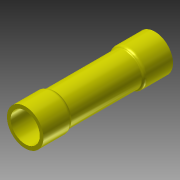
# Autodesk Inventor part: 12-10 double sided female tube yellow
Saved by Autodesk Inventor 2014 (Build 180170000, 170)
## iProperties
Created: 2013-07-20
Part Number: 12-10 double sided female tube yellow
Material: Generic
Document SubType Name: Modeling
Designer: Saville
Mass: 0.397287 g
Surface Area: 13.7194 cm^2
Volume: 0.397287 cm^3
Density: 1 g/cm^3
Appearance: Default
Author: Saville
Autodesk Inventor part; units mm, degrees
ref_plane "YZ Plane" through (0, 0, 0) normal (1, 0, 0) x (0, 1, 0)
ref_plane "XZ Plane" through (0, 0, 0) normal (0, 1, 0) x (-1, 0, 0)
ref_plane "XY Plane" through (0, 0, 0) normal (0, 0, 1) x (1, 0, 0)
sketch "Sketch1" plane through (0, 0, 0) normal (0, 0, 1) x (1, 0, 0)
  circle A0 centre (0, 0) radius 3.13055
  dimension "d0" = 6.2611
  constraints: 1 centre point, 1 coincident
  measures "d0" diameter of A0
extrude "Extrusion1" add sketch "Sketch1" along normal mid plane 24.7269
sketch "Sketch2" plane through (0, 0, 12.36345) normal (0, 0, 1) x (1, 0, 0)
  circle A0 centre (0, 0) radius 3.13055
  circle A1 centre (0, 0) radius 3.4798
  dimension "d3" = 6.9596
  constraints: 1 centre point, 1 coincident
  measures "d3" diameter of A1
extrude "Extrusion2" add sketch "Sketch2" against normal blind 5.461
fillet "Fillet1" radius 0.254 1 edges at (-3.1305, 0, 6.9024)
fillet "Fillet2" radius 0.762 1 edges at (-3.4798, 0, 6.9024)
mirror "Mirror1" about plane through (0, 0, 0) normal (0, 0, 1) of "Extrusion2", "Fillet1", "Fillet2"
shell "Shell1" thickness 0.6985 removed faces 2 at (0.449612, -0.769178, -12.36345) at (0.449612, -0.769178, 12.36345)
sketch "Sketch3" plane through (0, 0, 0) normal (1, 0, 0) x (0, 1, 0)
  line L0 (-3.4798, 7.415066) -> (-3.4798, 12.36345)
  line L1 (-3.4798, 12.36345) -> (-2.7813, 12.36345)
  line L2 (-2.7813, 12.36345) -> (-2.7813, 7.415066)
  line L3 (-2.43205, 6.64845) -> (-2.43205, -6.64845)
  line L4 (-2.7813, -7.415066) -> (-2.7813, -12.36345)
  line L5 (-2.7813, -12.36345) -> (-3.4798, -12.36345)
  line L6 (-3.4798, -12.36345) -> (-3.4798, -7.415066)
  arc A0 (-3.217862, -6.840104) -> (-3.13055, -6.64845) centre (-3.38455, -6.64845) ccw
  line L7 (-3.13055, -6.64845) -> (-3.13055, 6.64845)
  arc A1 (-3.13055, 6.64845) -> (-3.217862, 6.840104) centre (-3.38455, 6.64845) ccw
  arc A2 (3.217862, 6.840104) -> (3.13055, 6.64845) centre (3.38455, 6.64845) ccw
  line L8 (3.13055, 6.64845) -> (3.13055, -6.64845)
  arc A3 (3.13055, -6.64845) -> (3.217862, -6.840104) centre (3.38455, -6.64845) ccw
  line L9 (3.4798, -7.415066) -> (3.4798, -12.36345)
  line L10 (3.4798, -12.36345) -> (2.7813, -12.36345)
  line L11 (2.7813, -12.36345) -> (2.7813, -7.415066)
  line L12 (2.43205, -6.64845) -> (2.43205, 6.64845)
  line L13 (2.7813, 7.415066) -> (2.7813, 12.36345)
  line L14 (2.7813, 12.36345) -> (3.4798, 12.36345)
  line L15 (3.4798, 12.36345) -> (3.4798, 7.415066)
  line L16 (-2.43205, -7.41045) -> (-2.06375, -7.41045)
  line L17 (-2.06375, -7.41045) -> (-2.06375, 7.41045)
  line L18 (-2.06375, 7.41045) -> (-2.43205, 7.41045)
  line L19 (-2.43205, 7.41045) -> (-2.43205, -7.41045)
  line L20 (0, -17.30883) -> (0, 17.30883)
  arc A4 (-3.4798, 7.415066) -> (-3.217862, 6.840104) centre (-2.7178, 7.415066) ccw
  arc A5 (-2.7813, 7.415066) -> (-2.759472, 7.367153) centre (-2.7178, 7.415066) ccw
  arc A6 (-2.43205, 6.64845) -> (-2.759472, 7.367153) centre (-3.38455, 6.64845) ccw
  arc A7 (-2.759472, -7.367153) -> (-2.43205, -6.64845) centre (-3.38455, -6.64845) ccw
  arc A8 (-2.759472, -7.367153) -> (-2.7813, -7.415066) centre (-2.7178, -7.415066) ccw
  arc A9 (-3.217862, -6.840104) -> (-3.4798, -7.415066) centre (-2.7178, -7.415066) ccw
  arc A10 (3.217862, 6.840104) -> (3.4798, 7.415066) centre (2.7178, 7.415066) ccw
  arc A11 (3.4798, -7.415066) -> (3.217862, -6.840104) centre (2.7178, -7.415066) ccw
  arc A12 (2.7813, -7.415066) -> (2.759472, -7.367153) centre (2.7178, -7.415066) ccw
  arc A13 (2.43205, -6.64845) -> (2.759472, -7.367153) centre (3.38455, -6.64845) ccw
  arc A14 (2.759472, 7.367153) -> (2.43205, 6.64845) centre (3.38455, 6.64845) ccw
  arc A15 (2.759472, 7.367153) -> (2.7813, 7.415066) centre (2.7178, 7.415066) ccw
  point P0 (0, 0)
  dimension "d9" = 0.3683
  dimension "d10" = 0.762
  dimension "d11" = 0.762
  constraints: 8 end point, 2 parallel, 1 collinear, 1 horizontal, 1 perpendicular
  measures "d9" distance between parallel lines of L17 L19
  measures "d10" distance from line of L3.end L16
  measures "d11" distance from line of L18 L3.start
revolve "Revolution1" add sketch "Sketch3" angle 360 about axis through (0, 0, -10) along (0, 0, 1) separate body contours L19 L18 L17 L16 L3
chamfer "Chamfer1" distance 0.2032 angle 45 2 edges at (0, 2.0638, 7.4105) (0, 2.0637, -7.4105)
body "Solid1"
body "Solid2"
